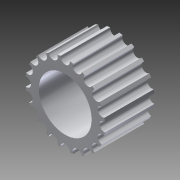
# Autodesk Inventor part: PulleyGT2x20Top
Saved by Autodesk Inventor 2016 (Build 200138000, 138)
## iProperties
Company: RobotDigg
Category: Hardware
Created: 2014-01-11
Part Number: PulleyGT2x20Top
Material: Aluminum 6061
Document SubType Name: Modeling
Designer: Jack
Density: 2.7 g/cm^3
Appearance: Aluminum - Flat
Mass: 0.919024 g
Surface Area: 7.13298 cm^2
Volume: 0.340379 cm^3
Vendor: RobotDigg
Catalog Web Link: http://www.robotdigg.com/product/23/GT2-Pulley-20-Teeth-8mm-Bore
Author: Jack
Title: GT2 Cut Pulley
Autodesk Inventor part; units mm, degrees
ref_plane "YZ Plane" through (0, 0, 0) normal (1, 0, 0) x (0, 1, 0)
ref_plane "XZ Plane" through (0, 0, 0) normal (0, 1, 0) x (-1, 0, 0)
ref_plane "XY Plane" through (0, 0, 0) normal (0, 0, 1) x (1, 0, 0)
ref_plane "Work Plane7" through (0, 6, 0) normal (0, 1, 0) x (1, 0, 0)
sketch "Sketch2" plane through (0, 6, 0) normal (0, 1, 0) x (1, 0, 0)
  line L0 (0.7, 6) -> (0.7, 5.9)
  line L1 (-0.7, 6) -> (-0.7, 5.9)
  arc A0 (-0.7, 5.9) -> (0.7, 5.9) centre (0, 5.9) ccw
  line L2 (-1.1884, 5.9227) -> (-1.1575, 5.8275)
  line L3 (-2.5198, 5.49) -> (-2.4889, 5.3949)
  arc A1 (-2.4889, 5.3949) -> (-1.1575, 5.8275) centre (-1.8232, 5.6112) ccw
  line L4 (-2.9604, 5.2656) -> (-2.9016, 5.1846)
  line L5 (-4.093, 4.4427) -> (-4.0342, 4.3618)
  arc A2 (-4.0342, 4.3618) -> (-2.9016, 5.1846) centre (-3.4679, 4.7732) ccw
  line L6 (-4.4427, 4.093) -> (-4.3618, 4.0342)
  line L7 (-5.2656, 2.9604) -> (-5.1846, 2.9016)
  arc A3 (-5.1846, 2.9016) -> (-4.3618, 4.0342) centre (-4.7732, 3.4679) ccw
  line L8 (-5.49, 2.5198) -> (-5.3949, 2.4889)
  line L9 (-5.9227, 1.1884) -> (-5.8275, 1.1575)
  arc A4 (-5.8275, 1.1575) -> (-5.3949, 2.4889) centre (-5.6112, 1.8232) ccw
  line L10 (-6, 0.7) -> (-5.9, 0.7)
  line L11 (-6, -0.7) -> (-5.9, -0.7)
  arc A5 (-5.9, -0.7) -> (-5.9, 0.7) centre (-5.9, 0) ccw
  line L12 (-5.9227, -1.1884) -> (-5.8275, -1.1575)
  line L13 (-5.49, -2.5198) -> (-5.3949, -2.4889)
  arc A6 (-5.3949, -2.4889) -> (-5.8275, -1.1575) centre (-5.6112, -1.8232) ccw
  line L14 (-5.2656, -2.9604) -> (-5.1846, -2.9016)
  line L15 (-4.4427, -4.093) -> (-4.3618, -4.0342)
  arc A7 (-4.3618, -4.0342) -> (-5.1846, -2.9016) centre (-4.7732, -3.4679) ccw
  line L16 (-4.093, -4.4427) -> (-4.0342, -4.3618)
  line L17 (-2.9604, -5.2656) -> (-2.9016, -5.1846)
  arc A8 (-2.9016, -5.1846) -> (-4.0342, -4.3618) centre (-3.4679, -4.7732) ccw
  line L18 (-2.5198, -5.49) -> (-2.4889, -5.3949)
  line L19 (-1.1884, -5.9227) -> (-1.1575, -5.8275)
  arc A9 (-1.1575, -5.8275) -> (-2.4889, -5.3949) centre (-1.8232, -5.6112) ccw
  line L20 (-0.7, -6) -> (-0.7, -5.9)
  line L21 (0.7, -6) -> (0.7, -5.9)
  arc A10 (0.7, -5.9) -> (-0.7, -5.9) centre (0, -5.9) ccw
  line L22 (1.1884, -5.9227) -> (1.1575, -5.8275)
  line L23 (2.5198, -5.49) -> (2.4889, -5.3949)
  arc A11 (2.4889, -5.3949) -> (1.1575, -5.8275) centre (1.8232, -5.6112) ccw
  line L24 (2.9604, -5.2656) -> (2.9016, -5.1846)
  line L25 (4.093, -4.4427) -> (4.0342, -4.3618)
  arc A12 (4.0342, -4.3618) -> (2.9016, -5.1846) centre (3.4679, -4.7732) ccw
  line L26 (4.4427, -4.093) -> (4.3618, -4.0342)
  line L27 (5.2656, -2.9604) -> (5.1846, -2.9016)
  arc A13 (5.1846, -2.9016) -> (4.3618, -4.0342) centre (4.7732, -3.4679) ccw
  line L28 (5.49, -2.5198) -> (5.3949, -2.4889)
  line L29 (5.9227, -1.1884) -> (5.8275, -1.1575)
  arc A14 (5.8275, -1.1575) -> (5.3949, -2.4889) centre (5.6112, -1.8232) ccw
  line L30 (6, -0.7) -> (5.9, -0.7)
  line L31 (6, 0.7) -> (5.9, 0.7)
  arc A15 (5.9, 0.7) -> (5.9, -0.7) centre (5.9, 0) ccw
  line L32 (5.9227, 1.1884) -> (5.8275, 1.1575)
  line L33 (5.49, 2.5198) -> (5.3949, 2.4889)
  arc A16 (5.3949, 2.4889) -> (5.8275, 1.1575) centre (5.6112, 1.8232) ccw
  line L34 (5.2656, 2.9604) -> (5.1846, 2.9016)
  line L35 (4.4427, 4.093) -> (4.3618, 4.0342)
  arc A17 (4.3618, 4.0342) -> (5.1846, 2.9016) centre (4.7732, 3.4679) ccw
  line L36 (4.093, 4.4427) -> (4.0342, 4.3618)
  line L37 (2.9604, 5.2656) -> (2.9016, 5.1846)
  arc A18 (2.9016, 5.1846) -> (4.0342, 4.3618) centre (3.4679, 4.7732) ccw
  line L38 (2.5198, 5.49) -> (2.4889, 5.3949)
  line L39 (1.1884, 5.9227) -> (1.1575, 5.8275)
  arc A19 (1.1575, 5.8275) -> (2.4889, 5.3949) centre (1.8232, 5.6112) ccw
  line L40 (-2.9604, 5.2656) -> (-2.5198, 5.49)
  line L41 (-1.1884, 5.9227) -> (-0.7, 6)
  line L42 (0.7, 6) -> (1.1884, 5.9227)
  line L43 (2.5198, 5.49) -> (2.9604, 5.2656)
  line L44 (4.093, 4.4427) -> (4.4427, 4.093)
  line L45 (5.2656, 2.9604) -> (5.49, 2.5198)
  line L46 (5.9227, 1.1884) -> (6, 0.7)
  line L47 (6, -0.7) -> (5.9227, -1.1884)
  line L48 (5.2656, -2.9604) -> (5.49, -2.5198)
  line L49 (4.4427, -4.093) -> (4.093, -4.4427)
  line L50 (2.9604, -5.2656) -> (2.5198, -5.49)
  line L51 (1.1884, -5.9227) -> (0.7, -6)
  line L52 (-0.7, -6) -> (-1.1884, -5.9227)
  line L53 (-2.5198, -5.49) -> (-2.9604, -5.2656)
  line L54 (-4.093, -4.4427) -> (-4.4427, -4.093)
  line L55 (-5.49, -2.5198) -> (-5.2656, -2.9604)
  line L56 (-5.9227, -1.1884) -> (-6, -0.7)
  line L57 (-6, 0.7) -> (-5.9227, 1.1884)
  line L58 (-5.49, 2.5198) -> (-5.2656, 2.9604)
  line L59 (-4.4427, 4.093) -> (-4.093, 4.4427)
  point P0 (0, 0)
  point P1 (-5.9, 0)
  dimension "d15" = 0.1
  dimension "d16" = 0.7
  dimension "d17" = 0.1
  dimension "d24" = 360
  dimension "d60" = 5.9
  dimension "d61" = 81
  constraints: 120 end point, 40 point on circle, 20 centre point, 20 coincident, 15 perpendicular, 2 tangent, 1 parallel, 1 vertical alignment, 182 other
  measures "d15" vertical distance of L0.start point (0, 5.9)
  measures "d16" radius of A0
  measures "d17" distance of L1.start L1.end
  measures "d60" distance of point (0, 0) A0.centre
  measures "d61" angle of L1 L41
extrude "Extrusion9" add sketch "Sketch2" along normal blind 7.5
sketch "Sketch11" plane through (0, 13.5, 0) normal (0, 1, 0) x (1, 0, 0)
  circle A0 centre (0, 0) radius 4
  dimension "d64" = 8
  constraints: 1 centre point, 1 coincident
  measures "d64" diameter of A0
extrude "Extrusion10" cut sketch "Sketch11" against normal up to next
body "Solid2"
